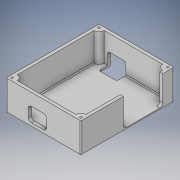
# Autodesk Inventor part: soporte_placa_techo
Saved by Autodesk Inventor 2019 (Build 230136000, 136)
## iProperties
Created: 2020-08-10
Part Number: soporte_placa_techo
Material: Generic
Document SubType Name: Modeling
Designer: Hugo Albarracin
Density: 1 g/cm^3
Appearance: Default
Author: Hugo Albarracin
Autodesk Inventor part; units mm, degrees
ref_plane "YZ Plane" through (0, 0, 0) normal (1, 0, 0) x (0, 1, 0)
ref_plane "XZ Plane" through (0, 0, 0) normal (0, 1, 0) x (-1, 0, 0)
ref_plane "XY Plane" through (0, 0, 0) normal (0, 0, 1) x (1, 0, 0)
sketch "Sketch1" plane through (0, 0, 0) normal (0, 1, 0) x (-1, 0, 0)
  line L0 (-37, 46) -> (37, 46)
  line L1 (37, 46) -> (37, -46)
  line L2 (37, -46) -> (-37, -46)
  line L3 (-37, -46) -> (-37, 46)
  line L4 (-37, 46) -> (37, -46) construction
  line L5 (37, 46) -> (-37, -46) construction
  point P0 (0, 0)
  dimension "d0" = 92
  dimension "d1" = 74
  constraints: 12 end point, 2 midpoint, 2 parallel, 1 horizontal, 1 perpendicular
  measures "d0" distance of L0.end L1.end
  measures "d1" distance of L1.end L2.end
extrude "Extrusion1" add sketch "Sketch1" along normal blind 2
sketch "Sketch2" plane through (0, 2, 0) normal (0, 1, 0) x (1, 0, 0)
  line L0 (34, -43) -> (29, -43) construction
  line L1 (-34, -43) -> (-34, -38) construction
  line L2 (-34, 43) -> (-29, 43) construction
  line L3 (34, 43) -> (34, 38) construction
  line L4 (34, -43) -> (-34, 43) construction
  line L5 (-34, -43) -> (34, 43) construction
  line L6 (-37, 46) -> (-37, -46) projected
  line L7 (37, 46) -> (-37, 46) projected
  line L8 (-37, -46) -> (37, -46) projected
  arc A0 (-34, 38) -> (-29, 43) centre (-34, 43) ccw
  arc A1 (29, 43) -> (34, 38) centre (34, 43) ccw
  arc A2 (-29, -43) -> (-34, -38) centre (-34, -43) ccw
  line L9 (-29, -43) -> (-34, -43) construction
  line L10 (-34, -38) -> (-34, 38)
  line L11 (34, -38) -> (34, -43) construction
  line L12 (29, -43) -> (-29, -43)
  arc A3 (34, -38) -> (29, -43) centre (34, -43) ccw
  line L13 (-34, 38) -> (-34, 43) construction
  line L14 (-29, 43) -> (29, 43)
  line L15 (29, 43) -> (34, 43) construction
  line L16 (34, 38) -> (34, -38)
  line L17 (-36.3721, 46) -> (36.3721, -46) construction
  line L18 (36.3721, 46) -> (-36.3721, -46) construction
  line L19 (37, 46) -> (-37, 46)
  line L20 (-37, 46) -> (-37, -46)
  line L21 (-37, -46) -> (37, -46)
  line L22 (37, -46) -> (37, 46)
  line L23 (37, 46) -> (-37, -46) construction
  line L24 (-37, 46) -> (37, -46) construction
  point P0 (0, 0)
  dimension "d4" = 3
  dimension "d5" = 3
  dimension "d17" = 5
  dimension "d18" = 5
  dimension "d19" = 5
  dimension "d20" = 5
  constraints: 44 end point, 20 parallel, 10 perpendicular, 8 point on circle, 6 midpoint, 4 centre point, 4 coincident, 4 horizontal, 2 point on line
  measures "d4" distance between parallel lines of L6 L1
  measures "d5" distance between parallel lines of L7 L2
  measures "d17" radius of A0
  measures "d18" radius of A1
  measures "d19" radius of A3
  measures "d20" radius of A2
extrude "Extrusion3" add sketch "Sketch2" along normal blind 28
sketch "Sketch3" plane through (0, 30, 0) normal (0, 1, 0) x (1, 0, 0)
  line L0 (-34, -38) -> (-34, 38) projected
  arc A0 (-34, 38) -> (-29, 43) centre (-34, 43) ccw projected
  line L1 (-29, 43) -> (29, 43) projected
  arc A1 (29, 43) -> (34, 38) centre (34, 43) ccw projected
  line L2 (34, 38) -> (34, -38) projected
  arc A2 (34, -38) -> (29, -43) centre (34, -43) ccw projected
  line L3 (29, -43) -> (-29, -43) projected
  arc A3 (-29, -43) -> (-34, -38) centre (-34, -43) ccw projected
  line L4 (-37, 46) -> (-37, -46) projected
  line L5 (-37, -46) -> (37, -46) projected
  line L6 (37, -46) -> (37, 46) projected
  line L7 (37, 46) -> (-37, 46) projected
  point P0 (0, 0)
hole "Hole1" at (34, 30, 43) at (-34, 30, 43) at (34, 30, -43) at (-34, 30, -43) direction (0, -1, 0) diameter 2 depth 25 tip angle 118
sketch "Sketch4" plane through (0, 0, 0) normal (0, -1, 0) x (1, 0, 0)
  line L0 (37, 46) -> (-37, 46) projected
  line L1 (-37, 46) -> (-37, -46) projected
  line L2 (-37, -46) -> (37, -46) projected
  line L3 (37, -46) -> (37, 46) projected
  line L4 (-25.5, -46) -> (-7.5, -46)
  line L5 (-7.5, -46) -> (-7.5, -34)
  line L6 (-7.5, -34) -> (-25.5, -34)
  line L7 (-25.5, -34) -> (-25.5, -46)
  line L8 (-25.5, -46) -> (-7.5, -34) construction
  line L9 (-25.5, -34) -> (-7.5, -46) construction
  line L10 (-16.5, -34) -> (-16.5, -46) construction
  line L11 (-25.5, -40) -> (-7.5, -40) construction
  point P0 (0, 0)
  dimension "d21" = 20.5
  dimension "d22" = 18
  dimension "d23" = 12
  constraints: 16 end point, 4 midpoint, 2 parallel, 1 horizontal, 1 perpendicular, 1 point on line
  measures "d21" distance between parallel lines of L1 L10
  measures "d22" distance of L5.end L6.end
  measures "d23" distance of L4.end L5.end
extrude "Extrusion4" cut sketch "Sketch4" against normal blind 14 contours L2 L7 L6 L5
sketch "Sketch5" plane through (37, 0, 46) normal (1, 0, 0) x (0, 0, -1)
  line L0 (81, 2) -> (42, 2)
  line L1 (42, 2) -> (42, 30)
  line L2 (42, 30) -> (81, 30)
  line L3 (81, 30) -> (81, 2)
  line L4 (92, 0) -> (0, 0) projected
  line L5 (92, 0) -> (92, 30) projected
  line L6 (0, 30) -> (92, 30) projected
  point P0 (46, 0)
  dimension "d26" = 2
  dimension "d27" = 11
  dimension "d28" = 50
  dimension "d29" = 0
  constraints: 8 end point, 2 parallel, 1 horizontal, 1 perpendicular
  measures "d26" distance between parallel lines of L0 L4
  measures "d27" distance between parallel lines of L3 L5
  measures "d28" distance between parallel lines of L1 L5
  measures "d29" distance between parallel lines of L6 L2
extrude "Extrusion5" cut sketch "Sketch5" against normal blind 5
fillet "Fillet1" radius 3 2 edges at (35.5, 2, -35) (35.5, 2, 4)
fillet "Fillet2" radius 2 4 edges at (-25.5, 1, -34) (-25.5, 14, -44.5) (-7.5, 14, -44.5) (-7.5, 1, -34)
fillet "Fillet3" radius 1 14 edges at (-31.25, 0, -46) (14.75, 0, -46) (37, 0, 0) (0, 0, 46) (-37, 0, 0) (-37, 15, -46) (37, 15, -46) (37, 15, 46) (-37, 15, 46) (-34, 2, 0) (0, 2, 43) (34, 2, 2.5) (34, 2, 21) (10.75, 2, -43)
sketch "Sketch6" plane through (-36, 1, 46) normal (0, 0, 1) x (1, 0, 0)
  line L0 (39, 17) -> (21, 17)
  line L1 (21, 17) -> (21, 3)
  line L2 (21, 3) -> (39, 3)
  line L3 (39, 3) -> (39, 17)
  line L4 (-1, 29) -> (-1, 0) projected
  line L5 (0, 29) -> (72, 29) projected
  point P0 (36, -1)
  dimension "d35" = 22
  dimension "d36" = 18
  dimension "d37" = 12
  dimension "d38" = 26
  constraints: 8 end point, 2 parallel, 1 horizontal, 1 perpendicular
  measures "d35" distance between parallel lines of L4 L1
  measures "d36" distance of L1.end L2.end
  measures "d37" distance between parallel lines of L5 L0
  measures "d38" distance between parallel lines of L5 L2
extrude "Extrusion6" cut sketch "Sketch6" against normal blind 5
fillet "Fillet4" radius 3 4 edges at (3, 4, 44.5) (-15, 4, 44.5) (3, 18, 44.5) (-15, 18, 44.5)
sketch "Sketch7" plane through (0, 0, 0) normal (0, -1, 0) x (1, 0, 0)
  line L0 (-21.569, 20.0079) -> (21.4213, 20.0079) construction
  line L1 (21.4213, 20.0079) -> (21.4213, -6.6351) construction
  line L2 (21.4213, -6.6351) -> (-21.569, -6.6351) construction
  line L3 (-21.569, -6.6351) -> (-21.569, 20.0079) construction
  spline S0 degree 2 poles (-5.5317, 13.8815) (-6.0617, 13.8815) (-6.8494, 14.1587) (-7.1265, 14.4358) knots 0 0 0 1 2 2 2
  spline S1 degree 2 poles (-7.1265, 14.4358) (-7.4426, 14.747) (-7.7002, 15.6222) (-7.7002, 16.264) knots 0 0 0 1 2 2 2
  line L4 (-7.7002, 16.264) -> (-7.7002, 20.0079)
  line L5 (-7.7002, 20.0079) -> (-6.9028, 20.0079)
  line L6 (-6.9028, 20.0079) -> (-6.9028, 16.264)
  spline S2 degree 2 poles (-6.9028, 16.264) (-6.9028, 15.8459) (-6.7959, 15.2818) (-6.6451, 15.0533) knots 0 0 0 1 2 2 2
  spline S3 degree 2 poles (-6.6451, 15.0533) (-6.4847, 14.8102) (-5.9304, 14.5622) (-5.5317, 14.5622) knots 0 0 0 1 2 2 2
  spline S4 degree 2 poles (-5.5317, 14.5622) (-5.1573, 14.5622) (-4.5738, 14.8102) (-4.4134, 15.0533) knots 0 0 0 1 2 2 2
  spline S5 degree 2 poles (-4.4134, 15.0533) (-4.2626, 15.2818) (-4.1557, 15.841) (-4.1557, 16.2446) knots 0 0 0 1 2 2 2
  line L7 (-4.1557, 16.2446) -> (-4.1557, 20.0079)
  line L8 (-4.1557, 20.0079) -> (-3.3583, 20.0079)
  line L9 (-3.3583, 20.0079) -> (-3.3583, 16.264)
  spline S6 degree 2 poles (-3.3583, 16.264) (-3.3583, 15.6368) (-3.6111, 14.7421) (-3.932, 14.4358) knots 0 0 0 1 2 2 2
  spline S7 degree 2 poles (-3.932, 14.4358) (-4.2189, 14.1538) (-4.9774, 13.8815) (-5.5317, 13.8815) knots 0 0 0 1 2 2 2
  spline S8 degree 2 poles (1.5769, 18.1992) (1.5769, 17.8102) (1.2998, 17.11) (1.0518, 16.8669) knots 0 0 0 1 2 2 2
  spline S9 degree 2 poles (1.0518, 16.8669) (0.7406, 16.5606) (-0.1006, 16.2446) (-0.7424, 16.2446) knots 0 0 0 1 2 2 2
  line L10 (-0.7424, 16.2446) -> (-1.4182, 16.2446)
  line L11 (-1.4182, 16.2446) -> (-1.4182, 14.0079)
  line L12 (-1.4182, 14.0079) -> (-2.2156, 14.0079)
  line L13 (-2.2156, 14.0079) -> (-2.2156, 20.0079)
  line L14 (-2.2156, 20.0079) -> (-0.7084, 20.0079)
  spline S10 degree 2 poles (-0.7084, 20.0079) (-0.1735, 20.0079) (0.5753, 19.8329) (0.8622, 19.6335) knots 0 0 0 1 2 2 2
  spline S11 degree 2 poles (0.8622, 19.6335) (1.1976, 19.405) (1.5769, 18.7) (1.5769, 18.1992) knots 0 0 0 1 2 2 2
  spline S12 degree 2 poles (0.7455, 18.1749) (0.7455, 18.4861) (0.5315, 18.9431) (0.3127, 19.089) knots 0 0 0 1 2 2 2
  spline S13 degree 2 poles (0.3127, 19.089) (0.1231, 19.2154) (-0.3826, 19.3175) (-0.757, 19.3175) knots 0 0 0 1 2 2 2
  line L15 (-0.757, 19.3175) -> (-1.4182, 19.3175)
  line L16 (-1.4182, 19.3175) -> (-1.4182, 16.9253)
  line L17 (-1.4182, 16.9253) -> (-0.8737, 16.9253)
  spline S14 degree 2 poles (-0.8737, 16.9253) (-0.3874, 16.9253) (0.2106, 17.0809) (0.4051, 17.2851) knots 0 0 0 1 2 2 2
  spline S15 degree 2 poles (0.4051, 17.2851) (0.585, 17.465) (0.7455, 17.888) (0.7455, 18.1749) knots 0 0 0 1 2 2 2
  line L18 (7.4797, 14.0079) -> (6.6822, 14.0079)
  line L19 (6.6822, 14.0079) -> (6.6822, 19.1765)
  line L20 (6.6822, 19.1765) -> (5.1166, 15.6611)
  line L21 (5.1166, 15.6611) -> (4.6304, 15.6611)
  line L22 (4.6304, 15.6611) -> (3.0793, 19.1765)
  line L23 (3.0793, 19.1765) -> (3.0793, 14.0079)
  line L24 (3.0793, 14.0079) -> (2.3354, 14.0079)
  line L25 (2.3354, 14.0079) -> (2.3354, 20.0079)
  line L26 (2.3354, 20.0079) -> (3.4245, 20.0079)
  line L27 (3.4245, 20.0079) -> (4.9221, 16.6676)
  line L28 (4.9221, 16.6676) -> (6.3711, 20.0079)
  line L29 (6.3711, 20.0079) -> (7.4797, 20.0079)
  line L30 (7.4797, 20.0079) -> (7.4797, 14.0079)
  line L31 (-12.3631, 4.1291) -> (-12.3631, 10.1291)
  line L32 (-12.3631, 10.1291) -> (-8.6095, 10.1291)
  line L33 (-8.6095, 10.1291) -> (-8.6095, 9.4192)
  line L34 (-8.6095, 9.4192) -> (-11.5657, 9.4192)
  line L35 (-11.5657, 9.4192) -> (-11.5657, 7.7758)
  line L36 (-11.5657, 7.7758) -> (-8.8088, 7.7758)
  line L37 (-8.8088, 7.7758) -> (-8.8088, 7.0659)
  line L38 (-8.8088, 7.0659) -> (-11.5657, 7.0659)
  line L39 (-11.5657, 7.0659) -> (-11.5657, 4.839)
  line L40 (-11.5657, 4.839) -> (-8.6095, 4.839)
  line L41 (-8.6095, 4.839) -> (-8.6095, 4.1291)
  line L42 (-8.6095, 4.1291) -> (-12.3631, 4.1291)
  line L43 (-6.334, 4.1291) -> (-6.334, 9.4192)
  line L44 (-6.334, 9.4192) -> (-8.3469, 9.4192)
  line L45 (-8.3469, 9.4192) -> (-8.3469, 10.1291)
  line L46 (-8.3469, 10.1291) -> (-3.5236, 10.1291)
  line L47 (-3.5236, 10.1291) -> (-3.5236, 9.4192)
  line L48 (-3.5236, 9.4192) -> (-5.5366, 9.4192)
  line L49 (-5.5366, 9.4192) -> (-5.5366, 4.1291)
  line L50 (-5.5366, 4.1291) -> (-6.334, 4.1291)
  spline S16 degree 2 poles (-1.2432, 4.0221) (-1.8947, 4.0221) (-2.8088, 4.2944) (-3.2124, 4.4889) knots 0 0 0 1 2 2 2
  line L51 (-3.2124, 4.4889) -> (-3.2124, 5.4905)
  line L52 (-3.2124, 5.4905) -> (-3.1541, 5.4905)
  spline S17 degree 2 poles (-3.1541, 5.4905) (-2.7602, 5.121) (-1.7635, 4.7126) (-1.3015, 4.7126) knots 0 0 0 1 2 2 2
  spline S18 degree 2 poles (-1.3015, 4.7126) (-0.6403, 4.7126) (0.0356, 5.262) (0.0356, 5.7142) knots 0 0 0 1 2 2 2
  spline S19 degree 2 poles (0.0356, 5.7142) (0.0356, 6.074) (-0.3194, 6.5213) (-0.7035, 6.6331) knots 0 0 0 1 2 2 2
  spline S20 degree 2 poles (-0.7035, 6.6331) (-0.9806, 6.7109) (-1.4426, 6.8179) (-1.7878, 6.9054) knots 0 0 0 1 2 2 2
  spline S21 degree 2 poles (-1.7878, 6.9054) (-2.099, 6.9881) (-2.59, 7.2361) (-2.7797, 7.4354) knots 0 0 0 1 2 2 2
  spline S22 degree 2 poles (-2.7797, 7.4354) (-2.9644, 7.6348) (-3.1686, 8.1696) (-3.1686, 8.5197) knots 0 0 0 1 2 2 2
  spline S23 degree 2 poles (-3.1686, 8.5197) (-3.1686, 9.249) (-2.0309, 10.2361) (-1.1508, 10.2361) knots 0 0 0 1 2 2 2
  spline S24 degree 2 poles (-1.1508, 10.2361) (-0.6451, 10.2361) (0.2495, 10.0367) (0.6336, 9.8471) knots 0 0 0 1 2 2 2
  line L53 (0.6336, 9.8471) -> (0.6336, 8.8941)
  line L54 (0.6336, 8.8941) -> (0.5753, 8.8941)
  spline S25 degree 2 poles (0.5753, 8.8941) (0.2884, 9.1566) (-0.6062, 9.5456) (-1.0973, 9.5456) knots 0 0 0 1 2 2 2
  spline S26 degree 2 poles (-1.0973, 9.5456) (-1.6516, 9.5456) (-2.3372, 9.0254) (-2.3372, 8.6024) knots 0 0 0 1 2 2 2
  spline S27 degree 2 poles (-2.3372, 8.6024) (-2.3372, 8.2231) (-1.9336, 7.7709) (-1.5544, 7.6688) knots 0 0 0 1 2 2 2
  spline S28 degree 2 poles (-1.5544, 7.6688) (-1.3015, 7.6007) (-0.5673, 7.4257) (-0.3242, 7.3528) knots 0 0 0 1 2 2 2
  spline S29 degree 2 poles (-0.3242, 7.3528) (0.2933, 7.1631) (0.867, 6.3998) (0.867, 5.8406) knots 0 0 0 1 2 2 2
  spline S30 degree 2 poles (0.867, 5.8406) (0.867, 5.4857) (0.5801, 4.8049) (0.3224, 4.5667) knots 0 0 0 1 2 2 2
  spline S31 degree 2 poles (0.3224, 4.5667) (0.0356, 4.3041) (-0.6938, 4.0221) (-1.2432, 4.0221) knots 0 0 0 1 2 2 2
  line L55 (3.7698, 4.1291) -> (1.4456, 4.1291)
  line L56 (1.4456, 4.1291) -> (1.4456, 4.7417)
  line L57 (1.4456, 4.7417) -> (2.209, 4.7417)
  line L58 (2.209, 4.7417) -> (2.209, 9.5165)
  line L59 (2.209, 9.5165) -> (1.4456, 9.5165)
  line L60 (1.4456, 9.5165) -> (1.4456, 10.1291)
  line L61 (1.4456, 10.1291) -> (3.7698, 10.1291)
  line L62 (3.7698, 10.1291) -> (3.7698, 9.5165)
  line L63 (3.7698, 9.5165) -> (3.0064, 9.5165)
  line L64 (3.0064, 9.5165) -> (3.0064, 4.7417)
  line L65 (3.0064, 4.7417) -> (3.7698, 4.7417)
  line L66 (3.7698, 4.7417) -> (3.7698, 4.1291)
  spline S32 degree 2 poles (9.4878, 7.1242) (9.4878, 6.3025) (8.8216, 4.98) (8.2625, 4.6105) knots 0 0 0 1 2 2 2
  spline S33 degree 2 poles (8.2625, 4.6105) (7.8054, 4.3236) (6.867, 4.1291) (6.1377, 4.1291) knots 0 0 0 1 2 2 2
  line L67 (6.1377, 4.1291) -> (4.7568, 4.1291)
  line L68 (4.7568, 4.1291) -> (4.7568, 10.1291)
  line L69 (4.7568, 10.1291) -> (6.1231, 10.1291)
  spline S34 degree 2 poles (6.1231, 10.1291) (6.9691, 10.1291) (7.9318, 9.8763) (8.2722, 9.6526) knots 0 0 0 1 2 2 2
  spline S35 degree 2 poles (8.2722, 9.6526) (8.8508, 9.2685) (9.4878, 7.9994) (9.4878, 7.1242) knots 0 0 0 1 2 2 2
  spline S36 degree 2 poles (8.6563, 7.134) (8.6563, 7.8244) (8.1993, 8.8017) (7.7471, 9.0789) knots 0 0 0 1 2 2 2
  spline S37 degree 2 poles (7.7471, 9.0789) (7.4262, 9.2685) (6.7017, 9.4387) (6.162, 9.4387) knots 0 0 0 1 2 2 2
  line L70 (6.162, 9.4387) -> (5.5542, 9.4387)
  line L71 (5.5542, 9.4387) -> (5.5542, 4.8195)
  line L72 (5.5542, 4.8195) -> (6.162, 4.8195)
  spline S38 degree 2 poles (6.162, 4.8195) (6.692, 4.8195) (7.4942, 4.9897) (7.82, 5.2182) knots 0 0 0 1 2 2 2
  spline S39 degree 2 poles (7.82, 5.2182) (8.2382, 5.5002) (8.6563, 6.4338) (8.6563, 7.134) knots 0 0 0 1 2 2 2
  line L73 (12.444, 4.1291) -> (10.1198, 4.1291)
  line L74 (10.1198, 4.1291) -> (10.1198, 4.7417)
  line L75 (10.1198, 4.7417) -> (10.8832, 4.7417)
  line L76 (10.8832, 4.7417) -> (10.8832, 9.5165)
  line L77 (10.8832, 9.5165) -> (10.1198, 9.5165)
  line L78 (10.1198, 9.5165) -> (10.1198, 10.1291)
  line L79 (10.1198, 10.1291) -> (12.444, 10.1291)
  line L80 (12.444, 10.1291) -> (12.444, 9.5165)
  line L81 (12.444, 9.5165) -> (11.6806, 9.5165)
  line L82 (11.6806, 9.5165) -> (11.6806, 4.7417)
  line L83 (11.6806, 4.7417) -> (12.444, 4.7417)
  line L84 (12.444, 4.7417) -> (12.444, 4.1291)
  point P0 (0, 0)
  constraints: 2 other
extrude "Extrusion7" cut sketch "Sketch7" against normal blind 1
body "Solid1"
